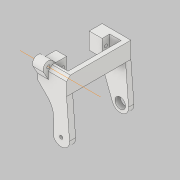
# Autodesk Inventor part: LegBase
Saved by Autodesk Inventor 2019.2 (Build 232265000, 265)
## iProperties
Created: 2019-01-14
Part Number: LegBase
Material: ABS-Kunststoff
Document SubType Name: Modeling
Designer: Lion
Density: 1.06 g/cm^3
Appearance: Weiß
Mass: 6.37954 g
Surface Area: 44.8159 cm^2
Volume: 6.01844 cm^3
Author: Lion
Autodesk Inventor part; units mm, degrees
ref_plane "YZ Plane" through (0, 0, 0) normal (1, 0, 0) x (0, 1, 0)
ref_plane "XZ Plane" through (0, 0, 0) normal (0, 1, 0) x (-1, 0, 0)
ref_plane "XY Plane" through (0, 0, 0) normal (0, 0, 1) x (1, 0, 0)
derived "BaseTop.ipt"
sketch "Skizze3" plane through (0, 0, 0) normal (0, 0, 1) x (1, 0, 0)
  circle A0 centre (-25.5, -32) radius 1 construction
  circle A1 centre (10, -35.5) radius 1 construction
  circle A2 centre (-22, 3.5) radius 1 construction
  circle A3 centre (13.5, 0) radius 1 construction
  line L0 (-28, 6) -> (16, 6)
  line L1 (16, 6) -> (16, -38)
  line L2 (16, -38) -> (-28, -38)
  line L3 (-28, -38) -> (-28, 6)
  circle A4 centre (-22, 3.5) radius 1
  circle A5 centre (13.5, 0) radius 1
  circle A6 centre (10, -35.5) radius 1
  circle A7 centre (-25.5, -32) radius 1
  line L4 (-16, -6) -> (4, -6)
  line L5 (4, -6) -> (4, -26)
  line L6 (4, -26) -> (-16, -26)
  line L7 (-16, -26) -> (-16, -6)
  line L8 (-11, -6) -> (-11, 6) construction
  line L9 (4, -11) -> (16, -11) construction
  line L10 (-1, -26) -> (-1, -38) construction
  line L11 (-16, -21) -> (-28, -21) construction
  circle A8 centre (-22, -15.5) radius 1.05
  line L12 (-22, -10) -> (-22, -23.5) construction
  line L13 (-12, -32) -> (1.5, -32) construction
  line L14 (10, -22) -> (10, -8.5) construction
  line L15 (-13.5, 0) -> (0, 0) construction
  circle A9 centre (10, -16.5) radius 1.05
  circle A10 centre (-5.5, 0) radius 1.05
  circle A11 centre (-6.5, -32) radius 1.05
  point P0 (-28, -38)
  point P1 (16, 6)
  point P2 (-16, -26)
  point P3 (4, -6)
sketch "Skizze2" plane through (0, 0, 0) normal (0, 0, 1) x (1, 0, 0)
  circle A0 centre (-5.5, 0) radius 1.05 construction
  line L0 (-5.5, 0) -> (-5.5, 25) construction
  line L1 (-21, 36) -> (10, 36) construction
  line L2 (10, 36) -> (10, 25) construction
  line L3 (10, 25) -> (-21, 25) construction
  line L4 (-21, 36) -> (10, 25) construction
  line L5 (10, 36) -> (-21, 25) construction
  line L6 (-5.5, 0) -> (-28, 6) construction
  line L7 (-2, 25) -> (-0.0178, 0.4425)
  line L8 (-21, 25) -> (-10.6339, -1.973)
  arc A1 (-10.6339, -1.973) -> (-0.0178, 0.4425) centre (-5.5, 0) ccw
  line L9 (-21, 25) -> (-21, 36)
  line L10 (-21, 36) -> (-5, 36)
  line L11 (-5, 36) -> (-2, 36)
  line L12 (-2, 36) -> (-2, 25)
  line L13 (-5, 25) -> (-21, 25)
  line L14 (-5, 25) -> (-2, 25)
  line L15 (-5, 25) -> (-5, 36)
  point P0 (0, 0)
  point P1 (-5.5, 30.5)
  point P2 (16, 6)
  dimension "d3" = 31
  dimension "d4" = 23.2863
  dimension "d5" = 25
  dimension "d6" = 11
  dimension "d9" = 5.5
  dimension "d65" = 16
  dimension "d66" = 3
  constraints: 32 end point, 5 perpendicular, 5 point on line, 3 midpoint, 2 point on circle, 2 tangent, 1 centre point, 1 collinear, 1 concentric, 1 horizontal, 1 parallel, 1 vertical
  measures "d3" distance of L3.end L2.end
  measures "d4" distance of L0.start L6.end
  measures "d5" distance of L0.end A0.centre
  measures "d6" distance between parallel lines of L1 L3
  measures "d9" radius of A1
  measures "d65" distance of L13.start L8.start
  measures "d66" distance between parallel lines of L12 L15
extrude "Extrusion1" add sketch "Skizze2" along normal blind 4
sketch "Skizze4" plane through (0, 0, 0) normal (0, 0, -1) x (-1, 0, 0)
  circle A0 centre (5.5, 0) radius 1.05 projected
  point P0 (0, 0)
extrude "Extrusion2" cut sketch "Skizze4" against normal blind 4
sketch "Skizze16" plane through (0, 0, 0) normal (0, 0, -1) x (-1, 0, 0)
  line L0 (5, 25) -> (2, 25) projected
  line L1 (2, 36) -> (2, 25) projected
  line L2 (5, 25) -> (5, 36) projected
  line L3 (5, 36) -> (2, 36) projected
  point P0 (0, 0)
extrude "Extrusion16" add sketch "Skizze16" along normal blind 35
sketch "Skizze5" plane through (0, 0, -35) normal (0, 0, -1) x (-1, 0, 0)
  line L0 (21, 25) -> (21, 36) projected
  line L1 (21, 36) -> (5, 36) projected
  line L2 (5, 36) -> (2, 36) projected
  line L3 (2, 36) -> (2, 25) projected
  line L4 (2, 25) -> (0.0178, 0.4425) projected
  arc A0 (0.0178, 0.4425) -> (10.6339, -1.973) centre (5.5, 0) ccw projected
  line L5 (21, 25) -> (10.6339, -1.973) projected
  point P0 (0, 0)
extrude "Extrusion4" add sketch "Skizze5" along normal blind 3.5
sketch "Skizze6" plane through (0, 0, -38.5) normal (0, 0, 1) x (1, 0, 0)
  circle A0 centre (-5.5, 0) radius 1
  arc A1 (-4.2877, 3.2834) -> (-8.555, 1.7078) centre (-5.5, 0) ccw
  line L0 (-5.5, 0) -> (-8.828, 14.6262) construction
  line L1 (-16.355, 12.9135) -> (-1.3009, 16.3388) construction
  circle A2 centre (-16.355, 12.9135) radius 15.4389 construction
  circle A3 centre (-1.3009, 16.3388) radius 15.4389 construction
  line L2 (-8.828, 14.6262) -> (-11.7944, 27.6634) construction
  circle A4 centre (-8.828, 14.6262) radius 2
  line L3 (-6.2928, 15.203) -> (-2.445, -1.7078) construction
  arc A5 (-3.4846, 2.8615) -> (-4.2877, 3.2834) centre (-5.5, 0) ccw
  arc A6 (-8.555, 1.7078) -> (-3.4846, 2.8615) centre (-5.5, 0) ccw
  line L4 (-11.3632, 14.0493) -> (-7.5154, -2.8615) construction
  line L5 (-10.7969, 14.2749) -> (-8.555, 1.7078)
  line L6 (-6.9009, 15.1614) -> (-3.4846, 2.8615)
  line L7 (-10.6339, -1.973) -> (-21, 25) construction
  line L8 (-2, 25) -> (-0.0178, 0.4425) construction
  dimension "d18" = 2
  dimension "d19" = 7
  dimension "d20" = 15
  dimension "d21" = 4
  dimension "d22" = 2.6
  constraints: 15 end point, 15 point on circle, 7 centre point, 4 coincident, 4 point on line, 3 symmetric about line, 2 tangent, 1 collinear, 1 midpoint, 1 parallel, 1 perpendicular
  measures "d18" diameter of A0
  measures "d19" diameter of A1
  measures "d20" distance of L0.start L0.end
  measures "d21" diameter of A4
  measures "d22" distance between parallel lines of L3 L0
extrude "LochHorn" cut sketch "Skizze6" along normal up to surface (3.5 mm away) contours A0 | A5 A6 A1
extrude "AussparungHorn" cut sketch "Skizze6" along normal blind 1.5 contours A0 | A5 A6 A1 | A1 L5 A4 L6 A5 | A4
sketch "Skizze8" plane through (0, 0, -35) normal (0, 0, 1) x (1, 0, 0)
  line L0 (-21, 25) -> (-21, 36) projected
  line L1 (-21, 36) -> (-5, 36) projected
  line L2 (-21, 36) -> (-12.5, 36)
  line L3 (-12.5, 36) -> (-12.5, 25)
  line L4 (-12.5, 25) -> (-21, 25)
  point P0 (0, 0)
  dimension "d69" = 8.5
  constraints: 6 end point, 1 parallel, 1 perpendicular, 1 point on line
  measures "d69" distance of L0.end L2.end
extrude "BlockUnten" add sketch "Skizze8" along normal blind 5
sketch "Skizze10" plane through (0, 0, 0) normal (0, 0, -1) x (-1, 0, 0)
  line L0 (21, 25) -> (21, 36) projected
  line L1 (21, 36) -> (5, 36) projected
  line L2 (21, 36) -> (14, 36)
  line L3 (14, 36) -> (14, 25)
  line L4 (14, 25) -> (21, 25)
  point P0 (0, 0)
  dimension "d70" = 7
  constraints: 6 end point, 2 perpendicular, 1 point on line
  measures "d70" distance of L0.end L2.end
extrude "BlockOben" add sketch "Skizze10" along normal blind 8
sketch "Skizze9" plane through (-21, 25, -38.5) normal (1, 0, 0) x (0, 0, -1)
  circle A0 centre (-6, 5.5) radius 1
  line L0 (0.05, 5.5) -> (-41.5, 5.5) construction
  circle A1 centre (-33, 5.5) radius 1.25
  line L1 (-8.5, 0) -> (-8.5, 11) construction
  line L2 (-30.5, 11) -> (-30.5, 0) construction
  line L3 (-42.5, 11) -> (0, 11) construction
  line L4 (-38.5, 0) -> (-3.5, 0) construction
  line L5 (-30.5, 0) -> (-8.5, 11) construction
  line L6 (-8.5, 0) -> (-30.5, 11) construction
  point P0 (-37.55, -25)
  point P1 (-19.5, 5.5)
  dimension "d33" = 2
  dimension "d39" = 2.5
  dimension "d71" = 2.5
  dimension "d72" = 2.5
  constraints: 6 end point, 3 point on line, 2 centre point, 1 midpoint, 1 perpendicular
  measures "d33" diameter of A0
  measures "d39" diameter of A1
  measures "d71" distance from line of L1 A0.centre
  measures "d72" distance from line of L2 A1.centre
extrude "ServoBefestigungLöcher" cut sketch "Skizze9" along normal up to surface (8.5 mm away)
sketch "Skizze15" plane through (0, 0, 4) normal (0, 0, 1) x (1, 0, 0)
  circle A0 centre (-21, 16.5) radius 6
  line L0 (-2, 36) -> (-21, 36) construction
  line L1 (-2, 25) -> (-2, 36) construction
  point P0 (0, 0)
  point P1 (-4, 36)
  point P2 (-2, 34)
  dimension "d62" = 12
  dimension "d75" = 19.5
  dimension "d76" = 19
  constraints: 1 centre point, 1 coincident
  measures "d62" diameter of A0
  measures "d75" distance from line of L0 point (-21, 16.5)
  measures "d76" distance from line of L1 point (-21, 16.5)
extrude "Extrusion15" cut sketch "Skizze15" against normal through all
sketch "Skizze17" plane through (0, 0, 4) normal (0, 0, 1) x (1, 0, 0)
  circle A0 centre (-5.5, 0) radius 1.05 construction
  line L0 (-5.5, 0) -> (-10.5, 0) construction
  line L1 (-10.5, 14.4636) -> (-10.5, -8.2816)
  line L2 (-10.5, -8.2816) -> (-21, -8.2816)
  line L3 (-21, 25) -> (-10.5, 14.4636)
  arc A1 (-16.3, 12.7704) -> (-20.0074, 22.4173) centre (-21, 16.5) ccw projected
  line L4 (-21, 25) -> (-21, -8.2816)
  point P0 (0, 0)
  dimension "d77" = 5
  constraints: 10 end point, 1 horizontal, 1 point on line, 1 tangent, 1 vertical
  measures "d77" distance of L0.start L0.end
extrude "Extrusion18" cut sketch "Skizze17" against normal up to surface (4 mm away)
fillet "Rundung5" radius 14 1 edges at (-10.5, 14.4636, 2)
sketch "Skizze22" plane through (-21, 25, -8) normal (-1, 0, 0) x (0, 0, 1)
  line L0 (12, 11) -> (12, 0) construction
  line L1 (0, 11) -> (12, 11) construction
  line L2 (12, 3.7704) -> (15.0625, 9.3056)
  line L3 (15.0625, 9.3056) -> (8.9375, 12.6944) construction
  line L4 (8.9375, 12.6944) -> (8, 11)
  line L5 (12, 11) -> (12, 11) construction
  arc A0 (15.0625, 9.3056) -> (8.9375, 12.6944) centre (12, 11) ccw
  line L6 (12, 3.7704) -> (12, 11)
  line L7 (12, 11) -> (8, 11)
  point P0 (8, -25)
  dimension "d112" = 7
  constraints: 12 end point, 3 perpendicular, 2 midpoint, 2 point on circle, 1 centre point, 1 collinear, 1 parallel, 1 point on line
  measures "d112" distance between parallel lines of L4 L2
extrude "Extrusion27" add sketch "Skizze22" against normal up to surface (7 mm away)
chamfer "Fase4" distance 2.5 angle 45 1 edges at (-8, 36, 4)
sketch "Skizze23" plane through (-21, 25, -8) normal (-1, 0, 0) x (0, 0, 1)
  circle A0 centre (12, 11) radius 1.05
  point P0 (8, -25)
  dimension "d124" = 2.1
  constraints: 1 centre point, 1 coincident
  measures "d124" diameter of A0
extrude "Extrusion28" cut sketch "Skizze23" against normal up to next
chamfer "Fase5" distance 1 angle 45 1 edges at (-17.5, 36, 0)
fillet "Rundung8" [suppressed]
